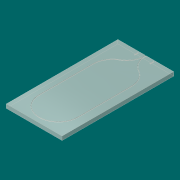
# Autodesk Inventor part: Scintillator Tile
Saved by Autodesk Inventor 2016 (Build 200138000, 138)
## iProperties
Created: 2015-08-14
Part Number: Scintillator Tile
Material: ABS Plastic
Document SubType Name: Modeling
Designer: Cosmic
Density: 1.06 g/cm^3
Appearance: Clear
Author: Cosmic
Autodesk Inventor part; units mm, degrees
ref_plane "YZ Plane" through (0, 0, 0) normal (1, 0, 0) x (0, 1, 0)
ref_plane "XZ Plane" through (0, 0, 0) normal (0, 1, 0) x (-1, 0, 0)
ref_plane "XY Plane" through (0, 0, 0) normal (0, 0, 1) x (1, 0, 0)
sketch "Sketch1" plane through (0, 0, 0) normal (0, 0, 1) x (1, 0, 0)
  line L0 (-72.5, -145) -> (72.5, -145)
  line L1 (72.5, -145) -> (72.5, 145)
  line L2 (72.5, 145) -> (-72.5, 145)
  line L3 (-72.5, 145) -> (-72.5, -145)
  line L4 (-72.5, -145) -> (72.5, 145) construction
  line L5 (72.5, -145) -> (-72.5, 145) construction
  point P0 (0, 0)
  dimension "d0" = 145
  dimension "d1" = 290
  constraints: 12 end point, 2 midpoint, 2 parallel, 1 horizontal, 1 perpendicular
  measures "d0" distance of L2.end L1.end
  measures "d1" distance of L1.end L0.end
extrude "Extrusion1" add sketch "Sketch1" along normal blind 10
sketch "Sketch6" plane through (0, 0, 10) normal (0, 0, 1) x (1, 0, 0)
  line L0 (-72.5, -145) -> (72.5, -145) projected
  line L1 (72.5, -145) -> (72.5, 145) projected
  line L2 (72.5, 145) -> (-72.5, 145) projected
  line L3 (-72.5, 145) -> (-72.5, -145) projected
  arc A0 (-49.5, -81.8686) -> (49.5, -81.8686) centre (0, -81.8686) ccw
  line L4 (-49.5, 58.1314) -> (-49.5, -81.8686)
  line L5 (49.5, 58.1314) -> (49.5, -81.8686)
  line L6 (-72.5, 142) -> (72.5, 142)
  line L7 (72.5, -145) -> (72.5, 145) projected
  line L8 (-72.5, -145) -> (72.5, -145) projected
  line L9 (0, -145) -> (0, 145)
  line L10 (72.5, 145) -> (-72.5, 145) projected
  arc A1 (-24.5516, 102.6045) -> (-1.3, 142) centre (-46.3, 142) ccw
  arc A2 (1.3, 142) -> (24.5516, 102.6045) centre (46.3, 142) ccw
  line L11 (-50.8, -81.8686) -> (-50.8, 58.1314)
  line L12 (50.8, 58.1314) -> (50.8, -81.8686)
  arc A3 (-50.8, -81.8686) -> (50.8, -81.8686) centre (0, -81.8686) ccw
  arc A4 (-23.9233, 101.4664) -> (0, 142) centre (-46.3, 142) ccw
  arc A5 (0, 142) -> (23.9233, 101.4664) centre (46.3, 142) ccw
  arc A6 (50.8, 58.1314) -> (24.5516, 102.6045) centre (0, 58.1314) ccw
  arc A7 (-24.5516, 102.6045) -> (-50.8, 58.1314) centre (0, 58.1314) ccw
  arc A8 (49.5, 58.1314) -> (23.9233, 101.4664) centre (0, 58.1314) ccw
  arc A9 (-23.9233, 101.4664) -> (-49.5, 58.1314) centre (0, 58.1314) ccw
  point P0 (0, 0)
  dimension "d80" = 3
  dimension "d83" = 90
  dimension "d84" = 90
  dimension "d86" = 1.3
  dimension "d87" = 1.3
  dimension "d88" = 1.3
  dimension "d89" = 99
  dimension "d90" = 49.5
  dimension "d91" = 49.5
  dimension "d92" = 1.3
  dimension "d93" = 1.3
  dimension "d94" = 1.3
  dimension "d114" = 140
  constraints: 20 point on circle, 12 end point, 10 centre point, 8 point on line, 6 tangent, 2 midpoint, 2 vertical, 1 perpendicular, 1 other
  measures "d80" distance between parallel lines of L6 L2
  measures "d83" diameter of A1
  measures "d84" diameter of A2
  measures "d86" distance between parallel lines of L4 L11
  measures "d87" radial gap between concentric circles of A4 A1
  measures "d88" radial gap between concentric circles of A5 A2
  measures "d89" distance between parallel lines of L4 L5
  measures "d90" radius of A9
  measures "d91" radius of A8
  measures "d92" radial gap between concentric circles of A9 A7
  measures "d93" radial gap between concentric circles of A6 A8
  measures "d94" distance between parallel lines of L5 L12
  measures "d114" distance of A0.centre A6.centre
extrude "Extrusion12" cut sketch "Sketch6" against normal blind 1.3 contours A3 L11 A7 A1 L6 A4 A9 L4 A0 L9 | L9 A0 L5 A8 A5 L6 A2 A6 L12 A3
sketch "Sketch8" plane through (0, 0, 10) normal (0, 0, 1) x (1, 0, 0)
  line L0 (72.5, 145) -> (-72.5, 145) projected
  line L1 (72.5, -145) -> (72.5, 145) projected
  line L2 (-72.5, -145) -> (72.5, -145) projected
  line L3 (-72.5, 145) -> (-72.5, -145) projected
  line L4 (-1.3, 145) -> (1.3, 145)
  line L5 (1.3, 145) -> (1.3, 135)
  line L6 (1.3, 135) -> (-1.3, 135)
  line L7 (-1.3, 135) -> (-1.3, 145)
  point P0 (0, 0)
  dimension "d59" = 2.6
  dimension "d60" = 10
  dimension "d61" = 71.2
  constraints: 8 end point, 2 parallel, 1 horizontal, 1 perpendicular, 1 point on line
  measures "d59" distance between parallel lines of L5 L7
  measures "d60" distance between parallel lines of L0 L6
  measures "d61" distance between parallel lines of L3 L7
extrude "Extrusion10" cut sketch "Sketch8" against normal up to surface (1.3 mm away) contours L5 L6 L7 L0
sketch "Sketch9" plane through (-72.5, 145, 0) normal (0, 1, 0) x (1, 0, 0)
  line L0 (71.2, -8.7) -> (73.8, -8.7)
  line L1 (145, -10) -> (73.8, -10)
  line L2 (145, 0) -> (145, -10)
  line L3 (145, 0) -> (0, 0)
  line L4 (0, 0) -> (0, -10)
  line L5 (96.4233, -10) -> (73.0322, -10)
  line L6 (75.525, -10) -> (69.475, -10)
  line L7 (69.475, -10) -> (69.475, -5.67)
  line L8 (69.475, -5.67) -> (75.525, -5.67)
  line L9 (75.525, -5.67) -> (75.525, -10)
  line L10 (72.5, -5.67) -> (72.5, -10)
  line L11 (73.0322, -10) -> (71.9678, -10)
  line L12 (71.2, -10) -> (71.2, -8.7)
  line L13 (73.8, -8.7) -> (73.8, -10)
  line L14 (71.2, -10) -> (0, -10)
  point P0 (72.5, 0)
  point P1 (76.3, -7)
  dimension "d64" = 4.33
  dimension "d65" = 6.05
  dimension "d66" = 72.5
  constraints: 28 end point, 2 midpoint, 2 parallel, 2 perpendicular, 1 horizontal, 4 other
  measures "d64" distance of L8.end L6.start
  measures "d65" distance of L7.end L8.end
  measures "d66" distance between parallel lines of L4 L10
extrude "Extrusion14" [suppressed]
fillet "Fillet2" radius 0.65 14 edges at (-7.5464, 119.1273, 8.7) (-43.7485, 83.9521, 8.7) (-50.8, -11.8686, 8.7) (0, -132.6686, 8.7) (50.8, -11.8686, 8.7) (43.7485, 83.9521, 8.7) (7.5464, 119.1273, 8.7) (42.6289, 83.2913, 8.7) (49.5, -11.8686, 8.7) (0, -131.3686, 8.7) (-49.5, -11.8686, 8.7) (-42.6289, 83.2913, 8.7) (-8.3257, 115.5114, 8.7) (8.3257, 115.5114, 8.7)
sketch "Sketch12" plane through (-72.5, 145, 0) normal (0, 1, 0) x (1, 0, 0)
  line L0 (71.2, -10) -> (71.2, -9.35) projected
  arc A0 (71.85, -8.7) -> (71.2, -9.35) centre (71.85, -9.35) ccw projected
  line L1 (71.85, -8.7) -> (73.15, -8.7) projected
  arc A1 (73.8, -9.35) -> (73.15, -8.7) centre (73.15, -9.35) ccw projected
  line L2 (73.8, -9.35) -> (73.8, -10) projected
  line L3 (145, -10) -> (73.8, -10) projected
  line L4 (145, 0) -> (145, -10) projected
  line L5 (145, 0) -> (0, 0) projected
  line L6 (0, 0) -> (0, -10) projected
  line L7 (71.2, -10) -> (0, -10) projected
  line L8 (145, -10) -> (73.8, -10) projected
  line L9 (145, 0) -> (0, 0) projected
  line L10 (72.5, 0) -> (72.5, -6)
  line L11 (72.5, -6) -> (92.5, -6)
  line L12 (72.5, -6) -> (52.5, -6)
  dimension "d103" = 20
  dimension "d104" = 20
  dimension "d105" = 4
  constraints: 6 end point, 1 collinear, 1 parallel, 1 perpendicular
  measures "d103" distance of L10.end L11.end
  measures "d104" distance of L10.end L12.end
  measures "d105" distance between parallel lines of L12 L7
hole "Hole2" at (-20, 145, 6) at (20, 145, 6) direction (0, -1, 0) diameter 2.459 depth 8.8 tip angle 118 thread size "M3x0.5" class "6H" standard "ISO Metric profile"
equation "\"d0\" = ScintillatorWidth"
equation "\"d1\" = ScintillatorHeight"
equation "\"d2\" = ScintillatorThickness"
equation "\"d80\" = ScintillatorEdgeClearence"
equation "\"d83\" = LoopSmallTrackDiameter"
equation "\"d84\" = LoopSmallTrackDiameter"
equation "\"d86\" = OpticalFiberDiameter + 2 * OpticalFiberClearence"
equation "\"d87\" = OpticalFiberDiameter + 2 * OpticalFiberClearence"
equation "\"d88\" = OpticalFiberDiameter + 2 * OpticalFiberClearence"
equation "\"d92\" = OpticalFiberDiameter + 2 * OpticalFiberClearence"
equation "\"d93\" = OpticalFiberDiameter + 2 * OpticalFiberClearence"
equation "\"d94\" = OpticalFiberDiameter + 2 * OpticalFiberClearence"
equation "\"d95\" = OpticalFiberDiameter + 2 * OpticalFiberClearence"
equation "\"d59\" = 4 * OpticalFiberClearence + 2 * OpticalFiberDiameter"
equation "\"d61\" = 0.5 * ScintillatorWidth - 2 * OpticalFiberClearence - OpticalFiberDiameter"
equation "\"d62\" = ShallowTrackDepth"
equation "\"d65\" = MPPCWidth + 2 * MPPCClearence"
equation "\"d66\" = 0.5 * ScintillatorWidth"
equation "\"d99\" = MPPCDepth"
equation "\"d5\" = OpticalFiberDiameter + 2 * OpticalFiberClearence"
equation "\"d21\" = d5"
equation "\"d22\" = d5"
equation "\"OpticalFiberDiameter\" = 1"
equation "\"ScintillatorThickness\" = 10"
equation "\"OpticalFiberClearence\" = 0.15"
equation "\"SmallTrackDiameter\" = 175"
equation "\"ScintillatorEdgeClearence\" = 3"
equation "\"ScintillatorWidth\" = 145"
equation "\"ScintillatorHeight\" = 290"
equation "\"ShallowTrackDepth\" = 1.3"
equation "\"MPPCClearence\" = 0.075"
equation "\"MPPCSensorClearence\" = 1.45"
equation "\"MPPCSensorOffsett\" = 2.105"
equation "\"MPPCWidth\" = 5.9"
equation "\"MPPCHeight\" = 6.55"
equation "\"FiberEdgeOffsett\" = 5"
equation "\"MPPCDepth\" = 1"
equation "\"LongFiberAngle\" = 30deg"
equation "\"ShortFiberAngle\" = 78deg"
equation "\"LoopLargeTrackRatio\" = 1.1"
equation "\"LoopSmallTrackDiameter\" = 90"
equation "\"FiberSensorClerence\" = 0.5"
equation "\"MountingScrewDepth\" = 4"
body "Solid1"
